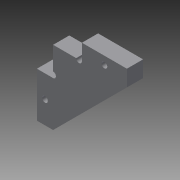
# Autodesk Inventor part: foot
Saved by Autodesk Inventor 2015 SP1 (Build 190203100, 203)
## iProperties
Created: 2015-04-10
Part Number: foot
Material: Generic
Document SubType Name: Modeling
Designer: Iain
Density: 1 g/cm^3
Appearance: Default
Author: Iain
Autodesk Inventor part; units mm, degrees
ref_plane "YZ Plane" through (0, 0, 0) normal (1, 0, 0) x (0, 1, 0)
ref_plane "XZ Plane" through (0, 0, 0) normal (0, 1, 0) x (-1, 0, 0)
ref_plane "XY Plane" through (0, 0, 0) normal (0, 0, 1) x (1, 0, 0)
sketch "Sketch1" plane through (0, 0, 0) normal (0, 1, 0) x (-1, 0, 0)
  line L0 (50, -50) -> (-50, -50)
  line L1 (-50, -50) -> (-50, 50)
  line L2 (-50, 50) -> (50, 50)
  line L3 (50, 50) -> (50, -50)
  point P0 (0, 0)
  point P1 (-50, 0)
  point P2 (0, -50)
  dimension "d0" = 100
  dimension "d1" = 100
  constraints: 8 end point, 2 midpoint, 2 parallel, 1 horizontal, 1 horizontal alignment, 1 perpendicular, 1 vertical alignment
  measures "d0" distance of L0.start L0.end
  measures "d1" distance of L2.end L0.start
extrude "Extrusion1" add sketch "Sketch1" along normal blind 18
sketch "Sketch2" plane through (0, 18, 0) normal (0, 1, 0) x (1, 0, 0)
  line L0 (-50, 50) -> (-32, 50) construction
  line L1 (50, 50) -> (-50, 50) construction
  line L2 (50, 50) -> (-50, 50) construction
  line L3 (-50, 50) -> (-50, -50) construction
  line L4 (-50, -50) -> (50, -50) construction
  line L5 (50, -50) -> (50, 50) construction
  line L6 (50, -50) -> (50, -32) construction
  line L7 (-32, 50) -> (50, -32)
  line L8 (50, -32) -> (50, 50)
  line L9 (50, 50) -> (-32, 50)
  point P0 (0, 0)
  point P1 (-41, 50)
  point P2 (0, 50)
  point P3 (-50, 0)
  point P4 (0, -50)
  point P5 (50, -41)
  point P6 (50, 0)
  dimension "d4" = 18
  dimension "d5" = 18
  constraints: 10 end point, 6 midpoint, 2 collinear, 2 horizontal alignment, 2 vertical alignment, 1 horizontal, 1 vertical
  measures "d4" distance of L0.start L0.end
  measures "d5" distance of L6.start L6.end
extrude "Extrusion2" cut sketch "Sketch2" against normal blind 18
sketch "Sketch3" plane through (0, 18, 0) normal (0, 1, 0) x (1, 0, 0)
  line L0 (-50, 0) -> (-32, 0)
  line L1 (-32, 0) -> (-32, -50)
  line L2 (-32, -50) -> (-50, -50)
  line L3 (-50, -50) -> (-50, 0)
  line L4 (50, -32) -> (-32, 50) projected
  line L5 (-32, 50) -> (-50, 50) projected
  line L6 (-50, 50) -> (-50, -50) projected
  line L7 (-50, -50) -> (50, -50) projected
  line L8 (50, -50) -> (50, -32) projected
  line L9 (-50, 50) -> (-50, -50) projected
  line L10 (-50, -32) -> (0, -32)
  line L11 (0, -32) -> (0, -50)
  line L12 (0, -50) -> (-50, -50)
  line L13 (-50, -50) -> (-50, -32)
  line L14 (-50, -50) -> (50, -50) projected
  point P0 (0, 0)
  point P1 (-41, -50)
  point P2 (-50, -25)
  point P3 (-50, 0)
  point P4 (-41, 0)
  point P5 (-50, 0)
  point P6 (-25, -50)
  point P7 (0, -50)
  point P8 (-50, -41)
  point P9 (0, -41)
  point P10 (0, -50)
  dimension "d8" = 18
  dimension "d9" = 18
  constraints: 16 end point, 10 midpoint, 4 parallel, 3 horizontal alignment, 3 vertical alignment, 2 horizontal, 2 perpendicular
  measures "d8" distance of L0.start L0.end
  measures "d9" distance of L12.end L10.start
extrude "Extrusion3" cut sketch "Sketch3" against normal blind 18 contours L0 L1 L10 L3 | L10 L1 L2 L3 | L10 L11 L7 L1
sketch "Sketch4" plane through (0, 18, 0) normal (0, 1, 0) x (1, 0, 0)
  line L0 (0, -32) -> (0, -50) projected
  line L1 (0, -50) -> (50, -50) projected
  line L2 (50, -50) -> (50, -32) projected
  line L3 (50, -32) -> (-32, 50) projected
  line L4 (-32, 50) -> (-50, 50) projected
  line L5 (-50, 50) -> (-50, 0) projected
  line L6 (-50, 0) -> (-32, 0) projected
  line L7 (-32, 0) -> (-32, -32) projected
  line L8 (-32, -32) -> (0, -32) projected
  point P0 (0, 0)
  point P1 (-32, -3.175)
  point P2 (-3.175, -32)
  point P3 (-16, -32)
  dimension "d12" = 3.175
  dimension "d13" = 3.175
  constraints: 1 horizontal alignment, 1 midpoint, 1 vertical alignment
  measures "d12" distance from line of L6 point (-32, -3.175)
  measures "d13" distance from line of L0 point (-3.175, -32)
hole "Hole1" at (-32, 18, 3.175) at (-3.175, 18, 32) direction (0, -1, 0) diameter 6.35 end through all
sketch "Sketch5" plane through (0, 18, 0) normal (0, 1, 0) x (1, 0, 0)
  arc A0 (-32, -6.35) -> (-32, 0) centre (-32, -3.175) ccw projected
  line L0 (-32, -6.35) -> (-32, -32) projected
  line L1 (-32, -32) -> (-6.35, -32) projected
  arc A1 (0, -32) -> (-6.35, -32) centre (-3.175, -32) ccw projected
  line L2 (0, -32) -> (0, -50) projected
  line L3 (0, -50) -> (50, -50) projected
  line L4 (50, -50) -> (50, -32) projected
  line L5 (50, -32) -> (-32, 50) projected
  line L6 (-32, 50) -> (-50, 50) projected
  line L7 (-50, 50) -> (-50, 0) projected
  line L8 (-50, 0) -> (-32, 0) projected
  point P0 (0, 0)
  point P1 (-41, 25)
  point P2 (25, -41)
  point P3 (-50, 25)
  point P4 (-41, 50)
  point P5 (0, -41)
  point P6 (25, -50)
  constraints: 4 midpoint, 2 horizontal alignment, 2 vertical alignment
hole "Hole2" at (-41, 18, -25) at (25, 18, 41) direction (0, -1, 0) diameter 6.35 end through all
equation "\"d0\" = legBaseWidth"
equation "\"d1\" = legBaseWidth"
equation "\"d2\" = plyThickness"
equation "\"d4\" = plyThickness"
equation "\"d5\" = d4"
equation "\"d6\" = plyThickness"
equation "\"d8\" = plyThickness"
equation "\"d9\" = d8"
equation "\"d10\" = plyThickness"
equation "\"d12\" = 0.5 * millDiameter"
equation "\"d13\" = 0.5 * millDiameter"
equation "\"d14\" = millDiameter"
equation "\"d21\" = millDiameter"
equation "\"plyThickness\" = 18"
equation "\"legHeight\" = 702"
equation "\"legBaseWidth\" = 100"
equation "\"millDiameter\" = 6.35"
equation "\"legTopTabHeight\" = 18"
equation "\"legTopSlotDepth\" = 49"
body "Solid1"
